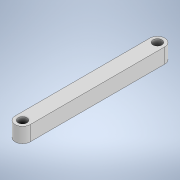
# Autodesk Inventor part: gripper1
Saved by Autodesk Inventor 2022 (Build 260153000, 153)
## iProperties
Created: 2022-01-07
Part Number: gripper1
Material: Generic
Document SubType Name: Modeling
Designer: nguye
Density: 1 g/cm^3
Appearance: Default
Author: nguye
Autodesk Inventor part; units mm, degrees
ref_plane "YZ Plane" through (0, 0, 0) normal (1, 0, 0) x (0, 1, 0)
ref_plane "XZ Plane" through (0, 0, 0) normal (0, 1, 0) x (-1, 0, 0)
ref_plane "XY Plane" through (0, 0, 0) normal (0, 0, 1) x (1, 0, 0)
sketch "Sketch1" plane through (0, 0, 0) normal (0, 1, 0) x (-1, 0, 0)
  line L0 (5, -2.5) -> (5, -47.5)
  line L1 (0, -47.5) -> (0, -2.5)
  arc A0 (5, -2.5) -> (0, -2.5) centre (2.5, -2.5) ccw
  arc A1 (0, -47.5) -> (5, -47.5) centre (2.5, -47.5) ccw
  circle A2 centre (2.5, -2.5) radius 1.5
  circle A3 centre (2.5, -47.5) radius 1.5
  point P0 (0, 0)
  dimension "d2" = 3
  dimension "d3" = 3
  constraints: 4 centre point, 4 end point, 4 point on circle, 2 coincident, 1 parallel
  measures "d2" diameter of A2
  measures "d3" diameter of A3
extrude "Extrusion1" add sketch "Sketch1" along normal blind 5
body "Solid1"
